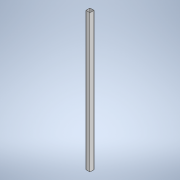
# Autodesk Inventor part: Mesa_base3
Saved by Autodesk Inventor 2021 (Build 250183000, 183)
## iProperties
Created: 2021-04-29
Part Number: Mesa_base3
Material: Genérico
Document SubType Name: Modeling
Designer: Admin
Density: 1 g/cm^3
Appearance: Valor por defecto
Author: Admin
Autodesk Inventor part; units mm, degrees
ref_plane "YZ Plane" through (0, 0, 0) normal (1, 0, 0) x (0, 1, 0)
ref_plane "XZ Plane" through (0, 0, 0) normal (0, 1, 0) x (-1, 0, 0)
ref_plane "XY Plane" through (0, 0, 0) normal (0, 0, 1) x (1, 0, 0)
sketch "Boceto1" plane through (0, 0, 0) normal (0, 1, 0) x (-1, 0, 0)
  line L0 (0, 0) -> (50, 0)
  line L1 (50, 0) -> (50, -50)
  line L2 (50, -50) -> (0, -50)
  line L3 (0, -50) -> (0, 0)
  line L4 (1.5, -48.5) -> (48.5, -48.5)
  line L5 (48.5, -48.5) -> (48.5, -1.5)
  line L6 (48.5, -1.5) -> (1.5, -1.5)
  line L7 (1.5, -1.5) -> (1.5, -48.5)
  line L8 (1.5, -48.5) -> (48.5, -1.5) construction
  line L9 (48.5, -48.5) -> (1.5, -1.5) construction
  point P0 (25, -25)
  dimension "d0" = 50
  dimension "d1" = 50
  dimension "d6" = 1.5
  dimension "d7" = 1.5
  dimension "d8" = 1.5
  dimension "d9" = 1.5
  constraints: 20 end point, 4 parallel, 2 horizontal, 2 midpoint, 2 perpendicular
  measures "d0" distance of L1.end L2.end
  measures "d1" distance of L0.end L1.end
  measures "d6" distance between parallel lines of L6 L0
  measures "d7" distance between parallel lines of L3 L7
  measures "d8" distance between parallel lines of L2 L4
  measures "d9" distance between parallel lines of L5 L1
extrude "Extrusión1" add sketch "Boceto1" along normal blind 1690.856
equation "\"d0\" = d1"
equation "\"d7\" = d6"
equation "\"d8\" = d6"
equation "\"d9\" = d6"
